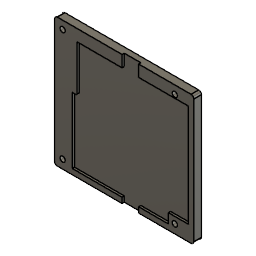
081326_AlignerAl (Autodesk Fusion 360 design; units mm, degrees)
part number: 2026-08-13-14-45-39-044
Autodesk Fusion 360 part; units mm, degrees
ref_plane "WorkPlane1" through (0, 0, 7) normal (0, 0, 1) x (1, 0, 0)
sketch "Base Plate Sketch" plane through (0, 0, 0) normal (0, 0, 1) x (1, 0, 0)
  line L0 (-58.1813, -58.7567) -> (67.977, -58.7567)
  line L1 (67.977, -58.7567) -> (67.977, 58.1813)
  line L2 (67.977, 58.1813) -> (-58.1813, 58.1813)
  line L3 (-58.1813, 58.1813) -> (-58.1813, -58.7567)
extrude "Base Plate" add sketch "Base Plate Sketch" along normal blind 7
fillet "Fillet1" radius 2.5 4 edges at (-58.1813, 58.1813, 3.5) (67.977, 58.1813, 3.5) (67.977, -58.7567, 3.5) (-58.1813, -58.7567, 3.5)
sketch "Wafer Nest Pocket Sketch" plane through (0, 0, 7) normal (0, 0, 1) x (1, 0, 0)
  line L0 (-42.023, -53.7567) -> (62.977, -53.7567)
  line L1 (62.977, -53.7567) -> (62.977, 47.704)
  line L2 (62.977, 47.704) -> (-42.023, 47.704)
  line L3 (-42.023, 47.704) -> (-42.023, -53.7567)
extrude "Wafer Nest Pocket" cut sketch "Wafer Nest Pocket Sketch" against normal blind 2
sketch "Front-Center Access Relief Sketch" plane through (0, 0, 7) normal (0, 0, 1) x (1, 0, 0)
  line L0 (2.977, -59.7567) -> (17.977, -59.7567)
  line L1 (17.977, -59.7567) -> (17.977, -50.7567)
  line L2 (17.977, -50.7567) -> (2.977, -50.7567)
  line L3 (2.977, -50.7567) -> (2.977, -59.7567)
extrude "Front-Center Access Relief" cut sketch "Front-Center Access Relief Sketch" against normal blind 2
sketch "Rear-Center Access Relief Sketch" plane through (0, 0, 7) normal (0, 0, 1) x (1, 0, 0)
  line L0 (2.977, 44.704) -> (17.977, 44.704)
  line L1 (17.977, 44.704) -> (17.977, 59.1812)
  line L2 (17.977, 59.1812) -> (2.977, 59.1812)
  line L3 (2.977, 59.1812) -> (2.977, 44.704)
extrude "Rear-Center Access Relief" cut sketch "Rear-Center Access Relief Sketch" against normal blind 2
sketch "X Datum Square Sketch (165 deg / 9:30)" plane through (0, 0, 7) normal (0, 0, 1) x (1, 0, 0)
  line L0 (-45.7852, 13.9038) -> (-37.7852, 13.9038)
  line L1 (-37.7852, 13.9038) -> (-37.7852, 6.9038)
  arc A0 (-38.7852, 5.9038) -> (-37.7852, 6.9038) centre (-38.7852, 6.9038) ccw
  line L2 (-38.7852, 5.9038) -> (-45.7852, 5.9038)
  line L3 (-45.7852, 5.9038) -> (-45.7852, 13.9038)
extrude "X Datum Square (165 deg / 9:30, rounded corner)" add sketch "X Datum Square Sketch (165 deg / 9:30)" against normal blind 2
sketch "Left Wall Flush Above X-Datum Sketch" plane through (0, 0, 7) normal (0, 0, 1) x (1, 0, 0)
  line L0 (-42.023, 13.9038) -> (-37.7852, 13.9038)
  line L1 (-37.7852, 13.9038) -> (-37.7852, 47.704)
  line L2 (-37.7852, 47.704) -> (-42.023, 47.704)
  line L3 (-42.023, 47.704) -> (-42.023, 13.9038)
extrude "Left Wall Flush Above X-Datum" add sketch "Left Wall Flush Above X-Datum Sketch" against normal blind 2
sketch "Front-Right Corner Clip (dowel) Sketch" plane through (0, 0, 7) normal (0, 0, 1) x (1, 0, 0)
  line L0 (44.9187, -53.7567) -> (62.977, -53.7567)
  line L1 (62.977, -53.7567) -> (62.977, -44.9187)
  line L2 (62.977, -44.9187) -> (44.9187, -44.9187)
  line L3 (44.9187, -44.9187) -> (44.9187, -53.7567)
extrude "Front-Right Corner Clip (dowel)" add sketch "Front-Right Corner Clip (dowel) Sketch" against normal blind 2
sketch "Outer Front Left Dowel Bore Sketch" plane through (0, 0, 7) normal (0, 0, 1) x (1, 0, 0)
  circle A0 centre (-50.8, -50.8) radius 2.3813
extrude "Outer Front Left Dowel Bore" cut sketch "Outer Front Left Dowel Bore Sketch" against normal blind 7
sketch "Outer Front Right Dowel Bore Sketch" plane through (0, 0, 7) normal (0, 0, 1) x (1, 0, 0)
  circle A0 centre (50.8, -50.8) radius 2.3813
extrude "Outer Front Right Dowel Bore" cut sketch "Outer Front Right Dowel Bore Sketch" against normal blind 7
sketch "Outer Rear Left Dowel Bore Sketch" plane through (0, 0, 7) normal (0, 0, 1) x (1, 0, 0)
  circle A0 centre (-50.8, 50.8) radius 2.3813
extrude "Outer Rear Left Dowel Bore" cut sketch "Outer Rear Left Dowel Bore Sketch" against normal blind 7
sketch "Outer Rear Right Dowel Bore Sketch" plane through (0, 0, 7) normal (0, 0, 1) x (1, 0, 0)
  circle A0 centre (50.8, 50.8) radius 2.3813
extrude "Outer Rear Right Dowel Bore" cut sketch "Outer Rear Right Dowel Bore Sketch" against normal blind 7
equation "gridPitch = 25.4 mm" comment "Table hole-grid pitch"
equation "indexMove = 50.8 mm" comment "Two-grid-space indexing move"
equation "outerPinPatternSpan = 101.6 mm" comment "Four-space outer pin span"
equation "dowelDiameter = 4.7625 mm" comment "3/16 in steel locating dowel diameter"
equation "dowelHoleDiameter = 4.7625 mm" comment "3/16 in reamed dowel bore"
equation "plateEdgeMargin = 5.0 mm" comment "Solid margin, plate edge to nearest feature"
equation "plateWidth = 126.15825000000001 mm" comment "Computed plate width (X)"
equation "plateHeight = 116.93795079844435 mm" comment "Computed plate height (Y)"
equation "baseThickness = 7.0 mm" comment "Base plate thickness"
equation "pocketDepth = 2.0 mm" comment "Wafer-nest pocket depth"
equation "nestClearanceSide = 2.5 mm" comment "Left/right pocket-wall clearance"
equation "nestClearanceRear = 4.0 mm" comment "Rear pocket-wall clearance"
equation "filletRadius = 2.5 mm" comment "Base-plate corner fillet radius"
equation "primaryFlatClearance = 0.175 mm" comment "Front wall forward of nominal flat"
equation "xDatumSize = 8.0 mm" comment "Square X-datum block side"
equation "nestReliefWidth = 15.0 mm" comment "Front/rear access relief width"
equation "nestOffsetX = 7.29 mm" comment "Nest X from pin-square center"
equation "nestOffsetY = -4.95 mm" comment "Nest Y from pin-square center"
